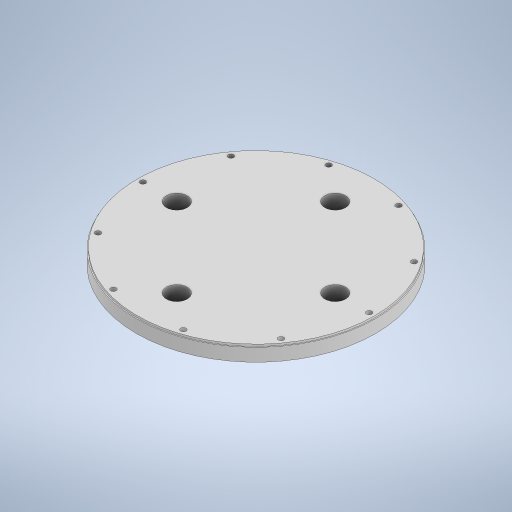
# Autodesk Inventor part: TampaBaixo
Saved by Autodesk Inventor 2024.2 (Build 282272000, 272)
## iProperties
Created: 2024-04-11
Part Number: TampaBaixo
Material: Generic
Document SubType Name: Modeling
Designer: 062210026
Density: 1 g/cm^3
Appearance: Default
Author: 062210026
Autodesk Inventor part; units mm, degrees
ref_plane "YZ Plane" through (0, 0, 0) normal (1, 0, 0) x (0, 1, 0)
ref_plane "XZ Plane" through (0, 0, 0) normal (0, 1, 0) x (-1, 0, 0)
ref_plane "XY Plane" through (0, 0, 0) normal (0, 0, 1) x (1, 0, 0)
sketch "Sketch1" plane through (0, 0, 0) normal (0, 1, 0) x (-1, 0, 0)
  circle A0 centre (-0.5297, 10.289) radius 21
  circle A1 centre (-80.0297, 10.289) radius 10.5
  circle A2 centre (-0.5297, -69.211) radius 10.5
  circle A3 centre (78.9703, 10.289) radius 10.5
  circle A4 centre (-0.5297, 89.789) radius 10.5
  circle A5 centre (-0.5297, 10.289) radius 120
  circle A6 centre (-0.5297, -69.211) radius 21
  circle A7 centre (78.9703, 10.289) radius 21
  circle A8 centre (-0.5297, 89.789) radius 21
  circle A9 centre (-80.0297, 10.289) radius 21
  circle A10 centre (-0.5297, 10.289) radius 119
  circle A11 centre (113.0263, 10.289) radius 2.75
  circle A12 centre (-0.5297, 10.289) radius 113.556
  circle A13 centre (91.339, 77.0355) radius 2.75
  circle A14 centre (34.561, 118.2872) radius 2.75
  circle A15 centre (-35.6205, 118.2872) radius 2.75
  circle A16 centre (-92.3985, 77.0355) radius 2.75
  circle A17 centre (-114.0857, 10.289) radius 2.75
  circle A18 centre (-92.3985, -56.4576) radius 2.75
  circle A19 centre (-35.6205, -97.7092) radius 2.75
  circle A20 centre (34.561, -97.7092) radius 2.75
  circle A21 centre (91.339, -56.4576) radius 2.75
  circle A22 centre (113.0263, 10.289) radius 6.12
  circle A23 centre (91.339, 77.0355) radius 6.12
  circle A24 centre (34.561, 118.2872) radius 6.12
  circle A25 centre (-35.6205, 118.2872) radius 6.12
  circle A26 centre (-92.3985, 77.0355) radius 6.12
  circle A27 centre (-114.0857, 10.289) radius 6.12
  circle A28 centre (-92.3985, -56.4576) radius 6.12
  circle A29 centre (-35.6205, -97.7092) radius 6.12
  circle A30 centre (34.561, -97.7092) radius 6.12
  circle A31 centre (91.339, -56.4576) radius 6.12
  point P0 (0, 0)
  dimension "d19" = 360
  dimension "d21" = 360
  constraints: 31 centre point, 8 coincident, 1 horizontal alignment, 44 other
extrude "Extrusion1" add sketch "Sketch1" against normal blind 15 contours A0 | A1 | A2 | A3 | A4 | A5 | A6 | A7 | A8 | A9 | A10 A22 A12 A11 | A10 A22 | A22 A12 A23 A10 | A10 A31 A12 A22 | A23 A12 A13 A10 | A10 A23 | A22 A12 A31 A30 A29 A28 A27 A26 A25 A24 A23 | A12 A11 A22 | A31 A10 | A10 A31 A12 A21 | A23 A12 A24 A10 | A12 A11 | A11 A12 | A23 A12 A13 | A10 A30 A12 A31 | A12 A21 A31 | A24 A12 A14 A10 | A10 A24 | A13 A12 | A12 A13 | A30 A10 | A10 A30 A12 A20 | A21 A12 | A12 A21 | A24 A12 A25 A10 | A24 A12 A14 | A10 A29 A12 A30 | A12 A20 A30 | A25 A12 A15 A10 | A10 A25 | A14 A12 | A12 A14 | A29 A10 | A10 A29 A12 A19 | A20 A12 | A12 A20 | A25 A12 A26 A10 | A25 A12 A15 | A10 A28 A12 A29 | A12 A19 A29 | A26 A12 A16 A10 | A10 A26 | A15 A12 | A12 A15 | A28 A10 | A10 A28 A12 A18 | A19 A12 | A12 A19 | A26 A12 A27 A10 | A26 A12 A16 | A10 A27 A12 A28 | A12 A18 A28 | A27 A12 A17 A10 | A10 A27 | A16 A12 | A12 A16 | A18 A12 | A12 A18 | A27 A12 A17 | A17 A12 | A12 A17
sketch "Sketch2" plane through (0.5297, 0, 10.289) normal (0, 1, 0) x (1, 0, 0)
  circle A0 centre (0, 0) radius 21
  circle A1 centre (-79.5, 0) radius 10.5
  circle A2 centre (0, -79.5) radius 10.5
  circle A3 centre (79.5, 0) radius 10.5
  circle A4 centre (0, 79.5) radius 10.5
  circle A5 centre (0, 0) radius 120
  circle A6 centre (0, -79.5) radius 21
  circle A7 centre (79.5, 0) radius 21
  circle A8 centre (0, 79.5) radius 21
  circle A9 centre (-79.5, 0) radius 21
  line L0 (0, 0) -> (113.556, 0)
  circle A10 centre (0, 0) radius 119
  circle A11 centre (113.556, 0) radius 2.75
  circle A12 centre (0, 0) radius 113.556
  circle A13 centre (91.8687, 66.7465) radius 2.75
  circle A14 centre (35.0907, 107.9982) radius 2.75
  circle A15 centre (-35.0907, 107.9982) radius 2.75
  circle A16 centre (-91.8687, 66.7465) radius 2.75
  circle A17 centre (-113.556, 0) radius 2.75
  circle A18 centre (-91.8687, -66.7465) radius 2.75
  circle A19 centre (-35.0907, -107.9982) radius 2.75
  circle A20 centre (35.0907, -107.9982) radius 2.75
  circle A21 centre (91.8687, -66.7465) radius 2.75
  circle A22 centre (113.556, 0) radius 6.12
  circle A23 centre (91.8687, 66.7465) radius 6.12
  circle A24 centre (35.0907, 107.9982) radius 6.12
  circle A25 centre (-35.0907, 107.9982) radius 6.12
  circle A26 centre (-91.8687, 66.7465) radius 6.12
  circle A27 centre (-113.556, 0) radius 6.12
  circle A28 centre (-91.8687, -66.7465) radius 6.12
  circle A29 centre (-35.0907, -107.9982) radius 6.12
  circle A30 centre (35.0907, -107.9982) radius 6.12
  circle A31 centre (91.8687, -66.7465) radius 6.12
  point P0 (-0.5297, 10.289)
  dimension "d43" = 360
  dimension "d45" = 360
  constraints: 31 centre point, 10 coincident, 2 end point, 1 horizontal alignment, 44 other
extrude "Extrusion2" cut sketch "Sketch2" against normal blind 2 contours A5 | A22 A10 | A10 A23 | A31 A10 | A10 A24 | A30 A10 | A10 A25 | A29 A10 | A10 A26 | A28 A10 | A10 A27
sketch "Sketch3" plane through (0.5297, 0, 10.289) normal (0, 1, 0) x (1, 0, 0)
  circle A0 centre (0, 0) radius 21
  circle A1 centre (-79.5, 0) radius 10.5
  circle A2 centre (0, -79.5) radius 10.5
  circle A3 centre (79.5, 0) radius 10.5
  circle A4 centre (0, 79.5) radius 10.5
  circle A5 centre (0, 0) radius 120
  circle A6 centre (0, -79.5) radius 21
  circle A7 centre (79.5, 0) radius 21
  circle A8 centre (0, 79.5) radius 21
  circle A9 centre (-79.5, 0) radius 21
  circle A10 centre (0, 0) radius 119
  circle A11 centre (113.556, 0) radius 2.75
  circle A12 centre (0, 0) radius 113.556
  circle A13 centre (91.8687, 66.7465) radius 2.75
  circle A14 centre (35.0907, 107.9982) radius 2.75
  circle A15 centre (-35.0907, 107.9982) radius 2.75
  circle A16 centre (-91.8687, 66.7465) radius 2.75
  circle A17 centre (-113.556, 0) radius 2.75
  circle A18 centre (-91.8687, -66.7465) radius 2.75
  circle A19 centre (-35.0907, -107.9982) radius 2.75
  circle A20 centre (35.0907, -107.9982) radius 2.75
  circle A21 centre (91.8687, -66.7465) radius 2.75
  circle A22 centre (113.556, 0) radius 6.12
  circle A23 centre (91.8687, 66.7465) radius 6.12
  circle A24 centre (35.0907, 107.9982) radius 6.12
  circle A25 centre (-35.0907, 107.9982) radius 6.12
  circle A26 centre (-91.8687, 66.7465) radius 6.12
  circle A27 centre (-113.556, 0) radius 6.12
  circle A28 centre (-91.8687, -66.7465) radius 6.12
  circle A29 centre (-35.0907, -107.9982) radius 6.12
  circle A30 centre (35.0907, -107.9982) radius 6.12
  circle A31 centre (91.8687, -66.7465) radius 6.12
  circle A32 centre (259.1085, 826.9411) radius 21
  circle A33 centre (259.1085, 747.4411) radius 10.5
  circle A34 centre (338.6085, 826.9411) radius 10.5
  circle A35 centre (179.6085, 826.9411) radius 10.5
  circle A36 centre (338.6085, 826.9411) radius 21
  circle A37 centre (259.1085, 747.4411) radius 21
  circle A38 centre (179.6085, 826.9411) radius 21
  circle A39 centre (372.6645, 826.9411) radius 2.75
  circle A40 centre (294.1992, 718.9429) radius 2.75
  circle A41 centre (224.0177, 718.9429) radius 2.75
  circle A42 centre (372.6645, 826.9411) radius 6.12
  circle A43 centre (294.1992, 718.9429) radius 6.12
  circle A44 centre (224.0177, 718.9429) radius 6.12
  circle A45 centre (350.9772, 760.1946) radius 6.12
  circle A46 centre (259.1085, 826.9411) radius 113.556
  circle A47 centre (259.1085, 826.9411) radius 120
  circle A48 centre (259.1085, 826.9411) radius 119
  circle A49 centre (350.9772, 760.1946) radius 2.75
  circle A50 centre (259.1085, 906.4411) radius 10.5
  circle A51 centre (350.9772, 893.6877) radius 2.75
  circle A52 centre (350.9772, 893.6877) radius 6.12
  circle A53 centre (259.1085, 906.4411) radius 21
  circle A54 centre (224.0177, 934.9393) radius 2.75
  circle A55 centre (294.1992, 934.9393) radius 2.75
  circle A56 centre (294.1992, 934.9393) radius 6.12
  circle A57 centre (167.2397, 760.1946) radius 2.75
  circle A58 centre (167.2397, 760.1946) radius 6.12
  circle A59 centre (224.0177, 934.9393) radius 6.12
  circle A60 centre (167.2397, 893.6877) radius 2.75
  circle A61 centre (167.2397, 893.6877) radius 6.12
  circle A62 centre (145.5525, 826.9411) radius 2.75
  circle A63 centre (145.5525, 826.9411) radius 6.12
  point P0 (-0.5297, 10.289)
  point P1 (-3.7436, -18.3778)
  point P2 (-3.7436, -18.3778)
  point P3 (-3.7436, -18.3778)
  point P4 (-3.7436, -18.3778)
  point P5 (258.5787, 837.2301)
  point P6 (255.3649, 808.5634)
  point P7 (255.3649, 808.5634)
  point P8 (255.3649, 808.5634)
  point P9 (255.3649, 808.5634)
  dimension "d52" = 360
  dimension "d53" = 360
  dimension "d58" = 360
  dimension "d59" = 360
  constraints: 62 centre point, 22 coincident, 2 horizontal alignment, 88 other
extrude "Extrusion3" cut sketch "Sketch3" against normal blind 30 contours A1 | A2 | A3 | A4 | A12 A11 | A11 A12 | A13 A12 | A12 A13 | A21 A12 | A12 A21 | A14 A12 | A12 A14 | A20 A12 | A12 A20 | A15 A12 | A12 A15 | A19 A12 | A12 A19 | A16 A12 | A12 A16 | A18 A12 | A12 A18 | A17 A12 | A12 A17
body "Solid1"
